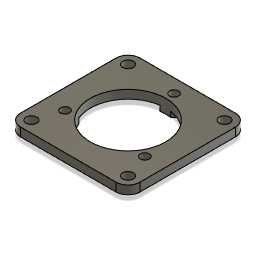
tweeter_adapter v2 (Autodesk Fusion 360 design; units mm, degrees)
Autodesk Fusion 360 part; units mm, degrees
note: some values were not read from the file. Set by a fixed rule: which sketch regions a step uses.
sketch "Sketch1" plane through (0, 0, 0) normal (0, 1, 0) x (1, 0, 0)
  line L0 (35, -35) -> (-35, -35)
  line L1 (-35, -35) -> (-35, 35)
  line L2 (-35, 35) -> (35, 35)
  line L3 (35, 35) -> (35, -35)
  line L4 (35, -35) -> (-35, 35) construction
  line L5 (-35, -35) -> (35, 35) construction
  dimension "d1" = 70
  dimension "d2" = 70
  constraint horizontal L0
  constraint perpendicular L0 L1
  constraint parallel L0 L2
  constraint parallel L1 L3
  constraint coincident L4 origin
  constraint coincident L5 origin
  measures "d1" distance of L1.end L2.end
  measures "d2" distance of L0.end L1.end
sketch "Sketch2" plane through (0, 0, 0) normal (0, 1, 0) x (1, 0, 0)
  line L0 (35, -35) -> (-35, 35)
  line L1 (28.2843, -28.2843) -> (-28.2843, -28.2843) construction
  line L2 (-28.2843, -28.2843) -> (-28.2843, 28.2843) construction
  line L3 (-28.2843, 28.2843) -> (28.2843, 28.2843) construction
  line L4 (28.2843, 28.2843) -> (28.2843, -28.2843) construction
  line L5 (28.2843, -28.2843) -> (-28.2843, 28.2843) construction
  line L6 (-28.2843, -28.2843) -> (28.2843, 28.2843) construction
  circle A0 centre (-28.2843, 28.2843) radius 3.125
  circle A1 centre (28.2843, 28.2843) radius 3.125
  circle A2 centre (-28.2843, -28.2843) radius 3.125
  circle A3 centre (28.2843, -28.2843) radius 3.125
  dimension "d6" = 80
  dimension "d7" = 6.25
  dimension "d12" = 6.25
  dimension "d13" = 6.25
  dimension "d14" = 6.25
  constraint horizontal L1
  constraint perpendicular L1 L2
  constraint parallel L1 L3
  constraint parallel L2 L4
  constraint coincident L5 origin
  constraint coincident L6 origin
  constraint coincident L2.end L3.start
  constraint coincident L3.end L4.start
  constraint coincident L1.end L2.start
  constraint coincident L1.start L4.end
  measures "d6" distance of L1.start L2.end
  measures "d7" diameter of A0
  measures "d12" diameter of A1
  measures "d13" diameter of A2
  measures "d14" diameter of A3
sketch "Sketch3" plane through (0, 0, 0) normal (0, 1, 0) x (1, 0, 0)
  circle A0 centre (0, 0) radius 22.1
  dimension "d15" = 44.2
  constraint coincident A0.centre origin
  measures "d15" diameter of A0
sketch "Sketch4" plane through (0, 0, 0) normal (0, 1, 0) x (1, 0, 0)
  circle A0 centre (0, 0) radius 27 construction
  circle A1 centre (0, 27) radius 2.625
  circle A2 centre (0, 27) radius 6
  circle A3 centre (-23.3827, -13.5) radius 2.625
  circle A4 centre (-23.3827, -13.5) radius 6
  circle A5 centre (23.3827, -13.5) radius 2.625
  circle A6 centre (23.3827, -13.5) radius 6
  dimension "d16" = 54
  dimension "d17" = 5.25
  dimension "d20" = 12
  dimension "d22" = 360
  constraint coincident A0.centre origin
  constraint coincident A0 A1.centre
  constraint concentric A1 A2
  measures "d16" diameter of A0
  measures "d17" diameter of A1
  measures "d20" diameter of A2
extrude "Extrude1" add sketch "Sketch1" against normal blind 5 makes body 1
extrude "Extrude4" add sketch "Sketch4" against normal blind 8 bodies 1
extrude "Extrude5" cut sketch "Sketch4" against normal up to surface (8 mm away) contours A1 | A3 | A5 bodies 1
fillet "Fillet1" radius 7 4 edges at (35, -2.5, 35) (35, -2.5, -35) (-35, -2.5, -35) (-35, -2.5, 35) on bodies 1
copy_body "Body->Comp1" bodies 1 removing the originals makes body 2 in component "Component"
extrude "Extrude1'" cut sketch "Sketch3" sketch "Sketch2" along normal up to surface of sketch 2 end surface through (0, -8, 0) normal (0, -1, 0) offset 0 bodies 2 in component "Component"
component "Component" placed x (1, 0, 0) y (0, 1, 0) z (0, 0, 1) at (0, 0, 0)
